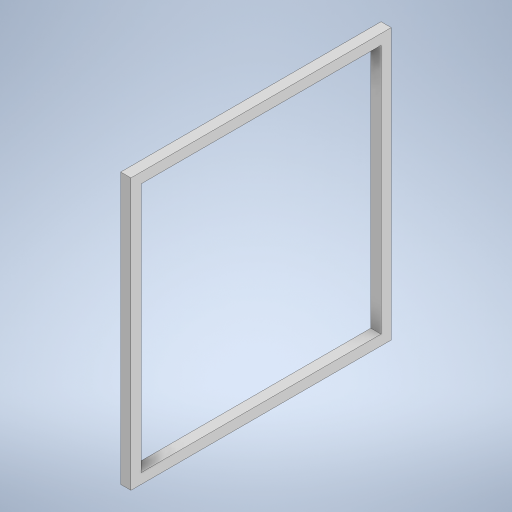
# Autodesk Inventor part: door1
Saved by Autodesk Inventor 2023.5 (Build 275446000, 446)
## iProperties
Created: 2025-04-17
Part Number: door1
Material: Generic
Document SubType Name: Modeling
Designer: LENOVO
Density: 1 g/cm^3
Appearance: Default
Author: LENOVO
Autodesk Inventor part; units mm, degrees
ref_plane "YZ Plane" through (0, 0, 0) normal (1, 0, 0) x (0, 1, 0)
ref_plane "XZ Plane" through (0, 0, 0) normal (0, 1, 0) x (-1, 0, 0)
ref_plane "XY Plane" through (0, 0, 0) normal (0, 0, 1) x (1, 0, 0)
sketch "Sketch1" plane through (0, 0, 0) normal (1, 0, 0) x (0, 1, 0)
  line L0 (0, 0) -> (530, 0)
  line L1 (530, 0) -> (530, -510)
  line L2 (530, -510) -> (0, -510)
  line L3 (0, -510) -> (0, 0)
  line L4 (510, -490) -> (510, -20)
  line L5 (510, -20) -> (20, -20)
  line L6 (20, -20) -> (20, -490)
  line L7 (20, -490) -> (510, -490)
  dimension "d0" = 530
  dimension "d1" = 510
  dimension "d2" = 20
  constraints: 16 end point, 4 parallel, 2 perpendicular, 1 horizontal, 3 other
  measures "d0" distance of L1.end L2.end
  measures "d1" distance of L0.end L1.end
  measures "d2" distance between parallel lines of L1 L4
extrude "Extrusion1" add sketch "Sketch1" along normal blind 20
body "Solid1"
